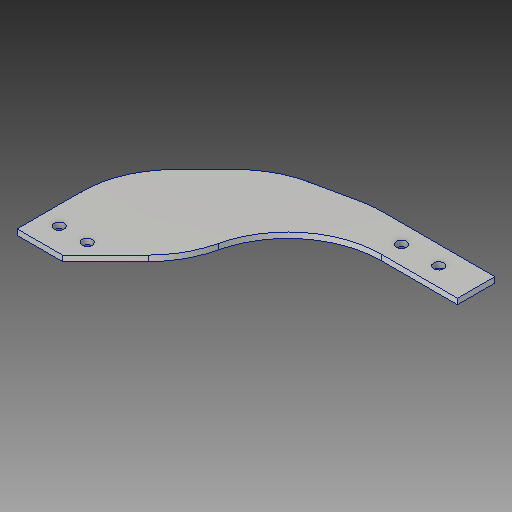
# Autodesk Inventor part: Support Plate
Saved by Autodesk Inventor 2019.4 (Build 234330000, 330)
## iProperties
Created: 2020-01-31
Part Number: Support Plate
Material: Aluminum 6061
Document SubType Name: Modeling
Designer: Mark
Mass: 51.6127 g
Surface Area: 142.492 cm^2
Volume: 19.1158 cm^3
Density: 2.7 g/cm^3
Appearance: Aluminum - Flat
Author: Mark
Autodesk Inventor part; units mm, degrees
ref_plane "YZ Plane" through (0, 0, 0) normal (1, 0, 0) x (0, 1, 0)
ref_plane "XZ Plane" through (0, 0, 0) normal (0, 1, 0) x (-1, 0, 0)
ref_plane "XY Plane" through (0, 0, 0) normal (0, 0, 1) x (1, 0, 0)
sketch "Sketch1" plane through (0, 0, 0) normal (0, 1, 0) x (-1, 0, 0)
  line L0 (150, 105.7) -> (125.7, 105.7)
  line L1 (0, 105.7) -> (0, 20) construction
  line L2 (0, 0) -> (150, 0)
  line L3 (150, 0) -> (150, 105.7)
  circle A0 centre (20, 10) radius 2.75
  circle A1 centre (40, 10) radius 2.75
  line L4 (0, 20) -> (40, 20)
  line L5 (40, 20) -> (125.7, 105.7)
  circle A2 centre (140, 93.2) radius 2.75
  circle A3 centre (125, 93.2) radius 2.75
  line L6 (125.7, 105.7) -> (0, 105.7) construction
  line L7 (0, 20) -> (0, 0)
  dimension "d0" = 150
  dimension "d1" = 105.7
  dimension "d2" = 5.5
  dimension "d3" = 5.5
  dimension "d4" = 20
  dimension "d5" = 20
  dimension "d6" = 10
  dimension "d7" = 10
  dimension "d8" = 135
  dimension "d9" = 20
  dimension "d10" = 40
  dimension "d11" = 5.5
  dimension "d12" = 5.5
  dimension "d13" = 12.5
  dimension "d14" = 12.5
  dimension "d15" = 10
  dimension "d16" = 25
  constraints: 16 end point, 4 centre point, 4 parallel, 4 perpendicular, 3 horizontal, 1 coincident
  measures "d0" distance of L2.end L2.start
  measures "d1" distance of L2.start L1.start
  measures "d2" diameter of A0
  measures "d3" diameter of A1
  measures "d4" distance of A0.centre A1.centre
  measures "d5" distance from line of L1 A0.centre
  measures "d6" distance from line of L2 A0.centre
  measures "d7" distance from line of L2 A1.centre
  measures "d8" angle of L0 L5
  measures "d9" distance between parallel lines of L2 L4
  measures "d10" distance of L1.end L4.end
  measures "d11" diameter of A2
  measures "d12" diameter of A3
  measures "d13" distance from line of L0 A3.centre
  measures "d14" distance from line of L0 A2.centre
  measures "d15" distance from line of L3 A2.centre
  measures "d16" distance from line of A3.centre L3
extrude "Extrusion1" add sketch "Sketch1" along normal blind 3
sketch "Sketch2" plane through (0, 3, 0) normal (0, 1, 0) x (1, 0, 0)
  line L0 (0, 0) -> (-150, 0) projected
  line L1 (-65.7, 0) -> (-108.3697, -9.0697)
  line L2 (-108.3697, -9.0697) -> (-150, -50.7)
  line L3 (-150, 0) -> (-150, -105.7) projected
  line L4 (-125.7, -105.7) -> (-40, -20) projected
  line L5 (-40, -20) -> (-65.7, -20)
  line L6 (-65.7, -20) -> (-90.7, -45)
  line L7 (-90.7, -45) -> (-90.7, -70.7)
  dimension "d19" = 45
  dimension "d21" = 12
  dimension "d22" = 65.7
  dimension "d23" = 135
  dimension "d24" = 135
  dimension "d25" = 55
  dimension "d26" = 35
  dimension "d28" = 25
  constraints: 10 end point, 3 point on line, 1 parallel
  measures "d19" angle of L3 L2
  measures "d21" angle of L0 L1
  measures "d22" distance of L0.start L1.start
  measures "d23" angle of L5 L6
  measures "d24" angle of L7 L6
  measures "d25" distance of L3.end L2.end
  measures "d26" horizontal distance of L4.start L7.end
  measures "d28" horizontal distance of L5.end L6.end
extrude "Extrusion2" cut sketch "Sketch2" against normal blind 3
fillet "Fillet1" radius 50 6 edges at (-65.7, 1.5, 0) (-108.3697, 1.5, 9.0697) (-65.7, 1.5, 20) (-90.7, 1.5, 45) (-90.7, 1.5, 70.7) (-150, 1.5, 50.7)
body "Solid1"
